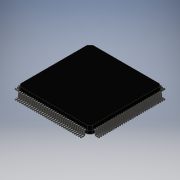
# Autodesk Inventor part: PI7CLQ128
Saved by Autodesk Inventor 2016 (Build 200138000, 138)
## iProperties
Created: 2017-03-03
Part Number: PI7CLQ128
Material: Generic
Document SubType Name: Modeling
Designer: jfixelle
Density: 1 g/cm^3
Appearance: Smooth - Black
Author: jfixelle
Autodesk Inventor part; units mm, degrees
ref_plane "XZ Plane" through (0, 0, 0) normal (0, 1, 0) x (-1, 0, 0)
ref_plane "XY Plane" through (0, 0, 0) normal (0, 0, 1) x (1, 0, 0)
sketch "Sketch1" plane through (0, 0, 0) normal (0, 1, 0) x (-1, 0, 0)
  line L0 (7, 7) -> (-7, 7)
  line L1 (-7, 7) -> (-7, -7)
  line L2 (-7, -7) -> (7, -7)
  line L3 (7, -7) -> (7, 7)
  point P0 (0, 0)
  dimension "d0" = 14
  dimension "d1" = 7
  dimension "d2" = 14
  dimension "d3" = 7
  constraints: 8 end point, 2 parallel, 1 horizontal, 1 perpendicular
  measures "d0" distance of L2.end L0.start
  measures "d1" distance from line of point (0, 0) L2
  measures "d2" distance of L1.end L2.end
  measures "d3" distance from line of point (0, 0) L3
extrude "Extrusion1" add sketch "Sketch1" along normal blind 1.45
chamfer "Chamfer1" distance 0.725 angle 10 1 edges at (-7, 1.45, 0) measured on face at (-7, 0.4833, -2.3333)
chamfer "Chamfer2" distance 0.725 angle 10 1 edges at (-7, 0, 0) measured on face at (-7, 0.2417, -2.3333)
chamfer "Chamfer3" distance 0.725 angle 10 1 edges at (0.0639, 0, -7) measured on face at (-2.2481, 0.4833, -7)
chamfer "Chamfer4" distance 0.725 angle 10 1 edges at (0.0639, 1.45, -7) measured on face at (-2.2907, 0.9667, -7)
chamfer "Chamfer5" distance 0.725 angle 10 1 edges at (7, 0, 0.0639) measured on face at (7, 0.9667, -2.2481)
chamfer "Chamfer6" distance 0.725 angle 10 1 edges at (7, 1.45, 0.0639) measured on face at (7, 0.9667, -2.2908)
chamfer "Chamfer7" distance 0.725 angle 10 1 edges at (0, 0, 7) measured on face at (2.2908, 0.9667, 7)
chamfer "Chamfer8" distance 0.725 angle 10 1 edges at (0.0001, 1.45, 7) measured on face at (-2.2907, 0.9667, 7)
chamfer "Chamfer9" distance 0.5 angle 45 8 edges at (-6.9361, 1.0876, 6.9361) (-6.9361, 0.3625, 6.9361) (-6.9361, 0.3625, -6.9361) (-6.9361, 1.0876, -6.9361) (6.9361, 0.3625, -6.9361) (6.9361, 1.0875, -6.9361) (6.9361, 0.3625, 6.9361) (6.9361, 1.0876, 6.9361)
ref_plane "Work Plane1" through (0.2, 0, 0) normal (1, 0, 0) x (0, 1, 0)
sketch "Sketch2" plane through (0.2, 0, 0) normal (1, 0, 0) x (0, 1, 0)
  line L0 (0.8535, 6.6067) -> (0.8535, 7.3388)
  line L1 (0.8535, 7.3388) -> (0.05, 7.4288)
  line L2 (0.05, 7.4288) -> (0.05, 8)
  line L3 (0.05, 8) -> (-0.15, 8)
  line L4 (-0.15, 8) -> (-0.15, 7.25)
  line L5 (-0.15, 7.25) -> (0.6535, 7.16)
  line L6 (0.6535, 7.16) -> (0.6535, 6.6067)
  line L7 (0.6535, 6.6067) -> (0.8535, 6.6067)
  line L8 (0, 6.3647) -> (0, -6.3647) projected
  line L9 (0, 0) -> (-0.4692, 0)
  line L10 (0.725, 7) -> (1.45, 6.8722) projected
  line L11 (0.725, 7) -> (0.6367, 7)
  dimension "d34" = 0.15
  dimension "d35" = 0.2
  dimension "d37" = 0.75
  dimension "d38" = 1
  dimension "d39" = 0.16
  dimension "d40" = 0.2
  dimension "d41" = 0.2
  constraints: 20 end point, 3 parallel, 3 perpendicular, 2 horizontal, 1 vertical
  measures "d34" distance between parallel lines of L4 L8
  measures "d35" distance between parallel lines of L4 L2
  measures "d37" distance of L3.end L4.end
  measures "d38" distance between parallel lines of L3 L11
  measures "d39" distance from line of L5.end L11
  measures "d40" distance between parallel lines of L0 L6
  measures "d41" distance between parallel lines of L5 L1
extrude "Extrusion2" add sketch "Sketch2" along normal mid plane 0.16
pattern_linear "Rectangular Pattern1" count 32 spacing 0.4 along (-1, 0, 0) of "Extrusion2" first direction both ways yes
pattern_circular "Circular Pattern1" count 4 over 360 about axis through (0, -10, 0) along (0, 1, 0) of "Extrusion2", "Rectangular Pattern1"
body "Solid1"
